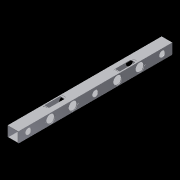
# Autodesk Inventor part: Side Box Tube
Saved by Autodesk Inventor 2014 SP1 (Build 180222100, 222)
## iProperties
Created: 2013-11-29
Part Number: Side Box Tube
Material: Aluminum 6061
Document SubType Name: Modeling
Designer: Rauhul Varma
Mass: 1048.75 g
Surface Area: 2556.04 cm^2
Volume: 386.992 cm^3
Density: 2.71 g/cm^3
Appearance: Aluminum - Flat
Author: Rauhul Varma
Autodesk Inventor part; units mm, degrees
ref_plane "YZ Plane" through (0, 0, 0) normal (1, 0, 0) x (0, 1, 0)
ref_plane "XZ Plane" through (0, 0, 0) normal (0, 1, 0) x (-1, 0, 0)
ref_plane "XY Plane" through (0, 0, 0) normal (0, 0, 1) x (1, 0, 0)
sketch "Sketch1" plane through (0, 0, 0) normal (0, 0, 1) x (1, 0, 0)
  line L0 (0, 0) -> (50.8, 0)
  line L1 (50.8, 0) -> (50.8, 50.8)
  line L2 (50.8, 50.8) -> (0, 50.8)
  line L3 (0, 50.8) -> (0, 0)
  line L4 (3.175, 3.175) -> (47.625, 3.175)
  line L5 (47.625, 3.175) -> (47.625, 47.625)
  line L6 (47.625, 47.625) -> (3.175, 47.625)
  line L7 (3.175, 47.625) -> (3.175, 3.175)
  dimension "d0" = 50.8
  dimension "d1" = 50.8
  dimension "d2" = 3.175
  dimension "d3" = 3.175
  dimension "d4" = 3.175
  dimension "d5" = 3.175
  constraints: 16 end point, 4 parallel, 2 horizontal, 2 perpendicular
  measures "d0" distance of L2.end L1.end
  measures "d1" distance of L1.end L0.end
  measures "d2" distance between parallel lines of L2 L6
  measures "d3" distance between parallel lines of L1 L5
  measures "d4" distance between parallel lines of L0 L4
  measures "d5" distance between parallel lines of L3 L7
extrude "Box Beam Profile" add sketch "Sketch1" along normal blind 736.6
ref_plane "Longitudal Midplane" through (0, 0, 368.3) normal (0, 0, 1) x (1, 0, 0)
ref_plane "Lateral Midplane" through (25.4, 0, 0) normal (-1, 0, 0) x (0, 0, 1)
sketch "Sketch2" plane through (0, 0, 0) normal (-1, 0, 0) x (0, 0, 1)
  line L0 (0, 50.8) -> (0, 0) projected
  line L1 (0, 0) -> (736.6, 0) projected
  line L2 (736.6, 50.8) -> (736.6, 0) projected
  line L3 (0, 50.8) -> (736.6, 50.8) projected
  line L4 (0, 25.4) -> (736.6, 25.4) construction
  line L5 (368.3, 50.8) -> (368.3, 0) construction
  circle A0 centre (368.3, 23.8125) radius 14.2875
  circle A1 centre (48.0396, 26.9875) radius 14.2875
  circle A2 centre (688.5604, 26.9875) radius 14.2875
  line L6 (368.4416, 9.5257) -> (688.702, 12.7007) construction
  line L7 (688.4188, 41.2743) -> (368.1584, 38.0993) construction
  line L8 (368.4416, 38.0993) -> (48.1812, 41.2743) construction
  line L9 (47.898, 12.7007) -> (368.1584, 9.5257) construction
  circle A3 centre (154.7931, 25.4) radius 19.05
  circle A4 centre (261.5465, 25.4) radius 19.05
  circle A5 centre (475.0535, 25.4) radius 19.05
  circle A6 centre (581.8069, 25.4) radius 19.05
  line L10 (688.5604, 50.8) -> (688.5604, 0) construction
  point P0 (25.4, 0)
  point P1 (711.2, 0)
  dimension "d9" = 28.575
  dimension "d11" = 320.2761
  dimension "d16" = 1.5875
  dimension "d17" = 1.5875
  dimension "d18" = 1.5875
  dimension "d19" = 38.1
  dimension "d20" = 38.1
  dimension "d21" = 38.1
  dimension "d22" = 38.1
  dimension "d23" = 106.7535
  dimension "d24" = 106.7535
  dimension "d25" = 106.7535
  constraints: 14 end point, 10 point on line, 8 point on circle, 8 tangent, 7 centre point, 4 midpoint, 3 symmetric about line, 2 equal radius, 1 perpendicular
  measures "d9" diameter of A0
  measures "d11" distance of A2.centre A0.centre
  measures "d16" distance from line of L4 A0.centre
  measures "d17" distance from line of L4 A2.centre
  measures "d18" distance from line of L4 A1.centre
  measures "d19" diameter of A3
  measures "d20" diameter of A4
  measures "d21" diameter of A5
  measures "d22" diameter of A6
  measures "d23" distance from line of L10 A6.centre
  measures "d24" distance from line of L5 A5.centre
  measures "d25" distance of A6.centre A5.centre
extrude "Through Cutouts" cut sketch "Sketch2" against normal through all contours A0 | A1 | A2 | A3 | A4 | A5 | A6
sketch "Sketch3" plane through (0, 0, 0) normal (-1, 0, 0) x (0, 0, 1)
  circle A0 centre (261.5465, 25.4) radius 19.05 projected
  circle A1 centre (154.7931, 25.4) radius 19.05 projected
  circle A2 centre (154.7931, 25.4) radius 22.225
  circle A3 centre (261.5465, 25.4) radius 22.225
  line L0 (261.5465, 25.4) -> (283.7715, 25.4)
  circle A4 centre (283.7715, 25.4) radius 4.7625
  line L1 (154.7931, 25.4) -> (132.5681, 25.4)
  circle A5 centre (132.5681, 25.4) radius 4.7625
  dimension "d28" = 44.45
  dimension "d30" = 44.45
  dimension "d31" = 9.525
  dimension "d71" = 9.525
  constraints: 4 coincident, 4 end point, 2 centre point, 2 horizontal, 2 horizontal alignment, 4 other
  measures "d31" diameter of A4
  measures "d71" diameter of A5
extrude "Plug Recesses" cut sketch "Sketch3" against normal blind 1.5875 contours L0 A4 A0 | L0 A3 A4 A0 | A0 A4 A3 L0 | A0 A4 L0 | A0 A4 A3 | A3 A4 | A1 A5 A2 | A5 L1 A1 | A1 L1 A2 A5 | A5 A2 L1 A1 | A1 L1 A5 | A2 A5
fillet "Fillet1" radius 3.175 2 edges at (0.7937, 30.1351, 283.2613) (0.7937, 20.6649, 283.2613)
mirror "Mirror1" about plane through (0, 0, 368.3) normal (0, 0, 1) of "Plug Recesses", "Fillet1"
mirror "Mirror2" about plane through (25.4, 0, 0) normal (-1, 0, 0) of "Plug Recesses", "Fillet1", "Mirror1"
sketch "Sketch4" plane through (0, 50.8, 0) normal (0, 1, 0) x (1, 0, 0)
  line L0 (50.8, 0) -> (0, 0) projected
  line L1 (0, 0) -> (0, -736.6) projected
  line L2 (50.8, -736.6) -> (0, -736.6) projected
  line L3 (50.8, 0) -> (50.8, -736.6) projected
  line L4 (25.4, 0) -> (25.4, -736.6) construction
  line L5 (0, -368.3) -> (50.8, -368.3) construction
  line L6 (6.7469, -350.8) -> (44.0531, -350.8) construction
  line L7 (44.0531, -350.8) -> (44.0531, -385.8) construction
  line L8 (44.0531, -385.8) -> (6.7469, -385.8) construction
  line L9 (6.7469, -385.8) -> (6.7469, -350.8) construction
  line L10 (26.6177, -385.8) -> (26.6177, 0) construction
  line L11 (41.6177, -385.8) -> (41.6177, 0) construction
  line L12 (-10.16, -48.0396) -> (60.96, -48.0396) projected
  line L13 (-10.16, -688.5604) -> (60.96, -688.5604) projected
  line L14 (22.9917, -170.0698) -> (45.2437, -170.0698)
  line L15 (45.2437, -170.0698) -> (45.2437, -246.2698)
  line L16 (45.2437, -246.2698) -> (22.9917, -246.2698)
  line L17 (22.9917, -246.2698) -> (22.9917, -170.0698)
  line L18 (0, -208.1698) -> (50.8, -208.1698) construction
  line L19 (0, -528.4302) -> (50.8, -528.4302) construction
  line L20 (27.0146, -490.3302) -> (4.7625, -490.3302)
  line L21 (4.7625, -490.3302) -> (4.7625, -566.5302)
  line L22 (4.7625, -566.5302) -> (27.0146, -566.5302)
  line L23 (27.0146, -566.5302) -> (27.0146, -490.3302)
  line L24 (42.0688, -170.0698) -> (42.0688, -246.2698)
  line L25 (26.1667, -170.0698) -> (26.1667, -246.2698)
  line L26 (24.5927, -166.8948) -> (43.6427, -166.8948)
  line L27 (43.6427, -166.8948) -> (43.6427, -160.5448)
  line L28 (43.6427, -160.5448) -> (24.5927, -160.5448)
  line L29 (24.5927, -160.5448) -> (24.5927, -166.8948)
  line L30 (24.5927, -249.4448) -> (43.6427, -249.4448)
  line L31 (43.6427, -249.4448) -> (43.6427, -255.7948)
  line L32 (43.6427, -255.7948) -> (24.5927, -255.7948)
  line L33 (24.5927, -255.7948) -> (24.5927, -249.4448)
  line L34 (6.3635, -487.1552) -> (25.4135, -487.1552)
  line L35 (25.4135, -487.1552) -> (25.4135, -480.8052)
  line L36 (25.4135, -480.8052) -> (6.3635, -480.8052)
  line L37 (6.3635, -480.8052) -> (6.3635, -487.1552)
  line L38 (6.3635, -569.7052) -> (25.4135, -569.7052)
  line L39 (25.4135, -569.7052) -> (25.4135, -576.0552)
  line L40 (25.4135, -576.0552) -> (6.3635, -576.0552)
  line L41 (6.3635, -576.0552) -> (6.3635, -569.7052)
  line L42 (15.8885, -566.5302) -> (15.8885, -490.3302) construction
  line L43 (34.1177, -170.0698) -> (34.1177, -246.2698) construction
  dimension "d38" = 35
  dimension "d39" = 37.3062
  dimension "d40" = 15
  dimension "d41" = 2.4354
  dimension "d43" = 5.5563
  dimension "d44" = 76.2
  dimension "d45" = 4.7625
  dimension "d47" = 76.2
  dimension "d52" = 3.175
  dimension "d53" = 0.451
  dimension "d54" = 0.451
  dimension "d55" = 3.175
  dimension "d56" = 22.2521
  dimension "d57" = 22.2521
  dimension "d73" = 6.35
  dimension "d74" = 6.35
  dimension "d75" = 6.35
  dimension "d76" = 6.35
  dimension "d77" = 19.05
  dimension "d78" = 19.05
  dimension "d79" = 19.05
  dimension "d80" = 19.05
  dimension "d81" = 3.175
  dimension "d82" = 3.175
  dimension "d83" = 3.175
  dimension "d84" = 3.175
  constraints: 76 end point, 14 parallel, 14 perpendicular, 12 point on line, 8 midpoint, 7 horizontal, 11 other
  measures "d38" distance between parallel lines of L8 L6
  measures "d39" distance between parallel lines of L7 L9
  measures "d40" distance between parallel lines of L11 L10
  measures "d41" distance between parallel lines of L11 L7
  measures "d43" distance between parallel lines of L3 L15
  measures "d44" distance between parallel lines of L16 L14
  measures "d45" distance between parallel lines of L1 L21
  measures "d47" distance between parallel lines of L22 L20
  measures "d52" distance between parallel lines of L15 L24
  measures "d53" distance between parallel lines of L10 L25
  measures "d54" distance between parallel lines of L24 L11
  measures "d55" distance between parallel lines of L25 L17
  measures "d56" distance of L15.end L16.end
  measures "d57" distance of L20.start L20.end
  measures "d73" distance of L40.end L38.start
  measures "d74" distance of L36.end L34.start
  measures "d75" distance of L28.end L26.start
  measures "d76" distance of L32.end L30.start
  measures "d77" distance of L38.start L38.end
  measures "d78" distance of L35.end L36.end
  measures "d79" distance of L31.end L32.end
  measures "d80" distance of L27.end L28.end
  measures "d81" distance between parallel lines of L14 L26
  measures "d82" distance between parallel lines of L16 L30
  measures "d83" distance between parallel lines of L34 L20
  measures "d84" distance between parallel lines of L22 L38
extrude "Belt Slots" cut sketch "Sketch4" against normal up to surface (3.175 mm away) contours L14 L25 L16 L17 | L14 L24 L16 L25 | L14 L15 L16 L24 | L23 L22 L21 L20
fillet "Fillet3" radius 3.175 8 edges at (45.2437, 49.2125, 170.0698) (45.2437, 49.2125, 246.2698) (22.9917, 49.2125, 246.2698) (22.9917, 49.2125, 170.0698) (4.7625, 49.2125, 490.3302) (27.0146, 49.2125, 490.3302) (27.0146, 49.2125, 566.5302) (4.7625, 49.2125, 566.5302)
fillet "Fillet4" radius 3.175 2 edges at (25.4, 0, 0) (25.4, 0, 736.6)
extrude "Extrusion7" cut sketch "Sketch4" against normal blind 1.5875 contours L29 L28 L27 L26 | L30 L31 L32 L33 | L37 L36 L35 L34 | L38 L39 L40 L41
fillet "Fillet5" radius 3.175 16 edges at (6.3635, 50.0062, 480.8052) (6.3635, 50.0062, 487.1552) (25.4135, 50.0062, 487.1552) (25.4135, 50.0062, 480.8052) (6.3635, 50.0062, 569.7052) (25.4135, 50.0062, 569.7052) (25.4135, 50.0062, 576.0552) (6.3635, 50.0062, 576.0552) (24.5927, 50.0062, 160.5448) (24.5927, 50.0062, 166.8948) (43.6427, 50.0062, 160.5448) (43.6427, 50.0062, 166.8948) (24.5927, 50.0062, 255.7948) (24.5927, 50.0062, 249.4448) (43.6427, 50.0062, 249.4448) (43.6427, 50.0062, 255.7948)
equation "\"d24\" = d25"
equation "\"d25\" = d23"
equation "\"d41\" = -0.666667 * d40 + 0.333333 * d39"
equation "\"d47\" = d44"
equation "\"d53\" = d54"
equation "\"d55\" = d52"
equation "\"d57\" = d56"
equation "\"d73\" = MagWidth"
equation "\"d74\" = MagWidth"
equation "\"d75\" = MagWidth"
equation "\"d76\" = MagWidth"
equation "\"d77\" = MagLength"
equation "\"d78\" = MagLength"
equation "\"d79\" = MagLength"
equation "\"d80\" = MagLength"
equation "\"MagWidth\" = 6.35"
equation "\"MagLength\" = 19.05"
body "Solid1"
